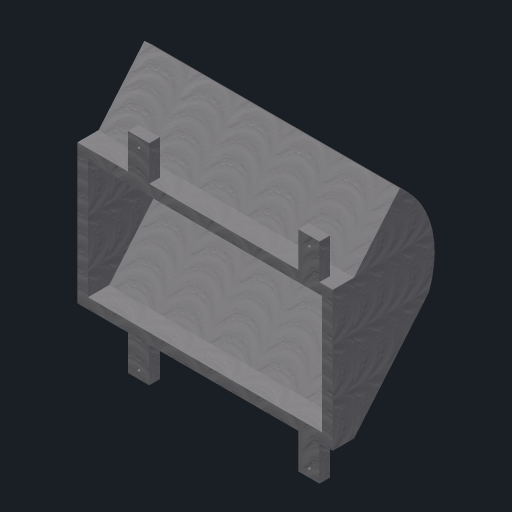
# Autodesk Inventor part: TOBOGAN_BASURA
Saved by Autodesk Inventor 2024.3 (Build 283343000, 343)
## iProperties
Created: 2024-06-23
Part Number: TOBOGAN_BASURA
Material: Steel, Mild, Welded
Document SubType Name: Modeling
Designer: Niler
Density: 7.85 g/cm^3
Appearance: Weld - Steel Mild
Author: Niler
Autodesk Inventor part; units mm, degrees
ref_plane "YZ Plane" through (0, 0, 0) normal (1, 0, 0) x (0, 1, 0)
ref_plane "XZ Plane" through (0, 0, 0) normal (0, 1, 0) x (-1, 0, 0)
ref_plane "XY Plane" through (0, 0, 0) normal (0, 0, 1) x (1, 0, 0)
sketch "Sketch1" plane through (0, 0, 0) normal (0, 0, 1) x (1, 0, 0)
  line L0 (-80, -90.5) -> (80, -90.5) construction
  line L1 (80, -90.5) -> (80, 90.5) construction
  line L2 (80, 90.5) -> (-80, 90.5) construction
  line L3 (-80, 90.5) -> (-80, -90.5) construction
  line L4 (-80, -90.5) -> (80, 90.5) construction
  line L5 (80, -90.5) -> (-80, 90.5) construction
  line L6 (-137.5, 65.5) -> (102.5, 65.5)
  line L7 (102.5, 65.5) -> (102.5, -65.5)
  line L8 (102.5, -65.5) -> (-137.5, -65.5)
  line L9 (-137.5, -65.5) -> (-137.5, 65.5)
  circle A0 centre (-80, 90.5) radius 1.65
  circle A1 centre (80, 90.5) radius 1.65
  circle A2 centre (-80, -90.5) radius 1.65
  circle A3 centre (80, -90.5) radius 1.65
  line L10 (92.5, 55.5) -> (-127.5, 55.5)
  line L11 (-127.5, 55.5) -> (-127.5, -55.5)
  line L12 (-127.5, -55.5) -> (92.5, -55.5)
  line L13 (92.5, -55.5) -> (92.5, 55.5)
  line L14 (-70, 65.5) -> (-90, 65.5)
  line L15 (-90, 65.5) -> (-90, 98.5)
  line L16 (-90, 98.5) -> (-70, 98.5)
  line L17 (-70, 98.5) -> (-70, 65.5)
  line L18 (90, 98.5) -> (70, 98.5)
  line L19 (70, 98.5) -> (70, 65.5)
  line L20 (70, 65.5) -> (90, 65.5)
  line L21 (90, 65.5) -> (90, 98.5)
  line L22 (90, -65.5) -> (70, -65.5)
  line L23 (70, -65.5) -> (70, -98.5)
  line L24 (70, -98.5) -> (90, -98.5)
  line L25 (90, -98.5) -> (90, -65.5)
  line L26 (-70, -65.5) -> (-90, -65.5)
  line L27 (-90, -65.5) -> (-90, -98.5)
  line L28 (-90, -98.5) -> (-70, -98.5)
  line L29 (-70, -98.5) -> (-70, -65.5)
  point P0 (0, 0)
  point P1 (102.5, 0)
  point P2 (-80, 98.5)
  point P3 (80, 65.5)
  point P4 (80, -98.5)
  point P5 (-80, -98.5)
  point P6 (70, -65.5)
  point P7 (-90, -65.5)
  point P8 (-90, 65.5)
  dimension "d0" = 181
  dimension "d1" = 160
  dimension "d3" = 3.3
  dimension "d4" = 10
  dimension "d5" = 240
  dimension "d6" = 22.5
  dimension "d15" = 25
  dimension "d16" = 20
  dimension "d21" = 20
  dimension "d22" = 33
  dimension "d23" = 20
  dimension "d25" = 20
  constraints: 60 end point, 17 parallel, 7 midpoint, 7 perpendicular, 6 horizontal, 4 centre point, 4 coincident, 4 point on line, 4 vertical alignment, 3 equal radius, 1 horizontal alignment, 3 other
  measures "d0" distance of L1.end L0.end
  measures "d1" distance of L1.end L2.end
  measures "d3" diameter of A0
  measures "d4" distance between parallel lines of L6 L10
  measures "d5" distance of L6.start L6.end
  measures "d6" distance from line of L7 A1.centre
  measures "d15" distance from line of L6 L2.end
  measures "d16" distance between parallel lines of L15 L17
  measures "d21" distance of L20.end L19.end
  measures "d22" distance of L19.end L18.end
  measures "d23" distance of L24.end L23.end
  measures "d25" distance of L28.end L28.start
extrude "Extrusion1" add sketch "Sketch1" against normal blind 20 contours L6 L7 L8 L9
extrude "Extrusion2" add sketch "Sketch1" against normal blind 10 contours L15 L16 L17 L6 | L8 L29 L28 L27 | L19 L18 L21 L6 | L8 L25 L24 L23
sketch "Sketch2" plane through (0, 0, 0) normal (1, 0, 0) x (0, 1, 0)
  line L0 (65.5, 0) -> (-65.5, 0) construction
  line L1 (65.5, 0) -> (65.5, -20) construction
  line L2 (-65.5, -20) -> (65.5, -20) construction
  line L3 (-65.5, 0) -> (-65.5, -20) construction
  line L4 (0, -20) -> (96.9885, -101.383)
  line L5 (-65.5, -20) -> (65.5, -20) projected
  point P0 (0, 0)
  dimension "d29" = 40
  constraints: 2 end point, 1 midpoint
  measures "d29" angle of L2 L4
sketch "Sketch3" plane through (0, 0, -20) normal (0, 0, -1) x (-1, 0, 0)
  line L0 (-102.5, -65.5) -> (137.5, -65.5) projected
  line L1 (137.5, -65.5) -> (137.5, 65.5) projected
  line L2 (137.5, 65.5) -> (-102.5, 65.5) projected
  line L3 (-102.5, 65.5) -> (-102.5, -65.5) projected
  line L4 (-92.5, -55.5) -> (-92.5, 55.5) projected
  line L5 (-92.5, 55.5) -> (127.5, 55.5) projected
  line L6 (127.5, 55.5) -> (127.5, -55.5) projected
  line L7 (127.5, -55.5) -> (-92.5, -55.5) projected
  point P0 (0, 0)
sweep "Sweep3" add profiles "Sketch3" path "Sketch2" separate body path curves L4
sketch "Sketch4" plane through (-137.5, -65.5, -20) normal (-1, 0, 0) x (0, 0, 1)
  line L0 (0, 0) -> (0, 131) projected
  line L1 (0, 131) -> (-81.383, 227.9885) projected
  line L2 (-81.383, 96.9885) -> (-81.383, 227.9885) projected
  line L3 (0, 0) -> (-81.383, 96.9885) projected
  arc A0 (-42.91, 182.1381) -> (-70.435, 83.9412) centre (11.7677, 113.8556) ccw
  point P0 (20, 65.5)
  constraints: 2 point on circle, 2 point on line, 1 centre point
extrude "Extrusion3" cut sketch "Sketch4" against normal through all contours L3 L2 L1 A0 bodies 2
body "Solid1"
body "Solid4"
